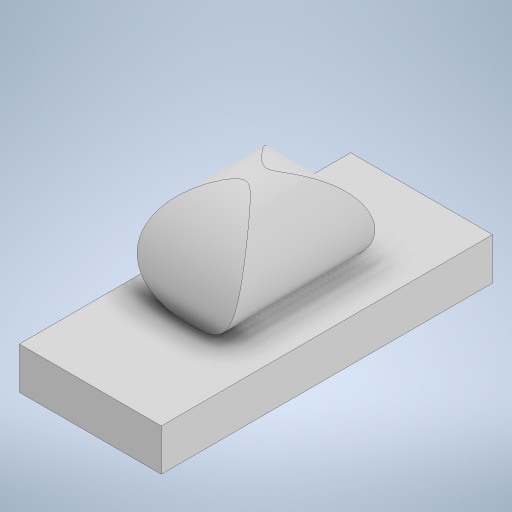
# Autodesk Inventor part: ball transfer unit
Saved by Autodesk Inventor 2023 (Build 270158000, 158)
## iProperties
Created: 2022-11-09
Part Number: ball transfer unit
Material: Generic
Document SubType Name: Modeling
Designer: cheng
Density: 1 g/cm^3
Appearance: Default
Author: cheng
Autodesk Inventor part; units mm, degrees
ref_plane "YZ Plane" through (0, 0, 0) normal (1, 0, 0) x (0, 1, 0)
ref_plane "XZ Plane" through (0, 0, 0) normal (0, 1, 0) x (-1, 0, 0)
ref_plane "XY Plane" through (0, 0, 0) normal (0, 0, 1) x (1, 0, 0)
sketch "Sketch1" plane through (0, 0, 0) normal (0, 1, 0) x (-1, 0, 0)
  line L0 (15, -35) -> (-15, -35)
  line L1 (-15, -35) -> (-15, 35)
  line L2 (-15, 35) -> (15, 35)
  line L3 (15, 35) -> (15, -35)
  line L4 (15, -35) -> (-15, 35) construction
  line L5 (-15, -35) -> (15, 35) construction
  point P0 (0, 0)
  dimension "d0" = 30
  dimension "d1" = 70
  constraints: 12 end point, 2 midpoint, 2 parallel, 1 horizontal, 1 perpendicular
  measures "d0" distance of L0.start L0.end
  measures "d1" distance of L2.end L0.start
extrude "Extrusion1" add sketch "Sketch1" along normal blind 30
sketch "Sketch2" plane through (15, 0, 35) normal (1, 0, 0) x (0, 0, -1)
  circle A0 centre (35, 15.1375) radius 14.909
  line L0 (0, 0) -> (0, 30) projected
  line L1 (0, 8.8455) -> (70, 8.8455)
  line L2 (0, 30) -> (70, 30) projected
  line L3 (0, 0) -> (70, 0) projected
  line L4 (70, 0) -> (70, 30) projected
  point P0 (35, 0)
  point P1 (36.1767, 30)
  point P2 (21.4837, 8.8455)
  point P3 (33.8233, 30)
  point P4 (48.5163, 8.8455)
  constraints: 2 end point, 2 point on line, 1 centre point, 1 horizontal, 1 perpendicular
extrude "Extrusion2" cut sketch "Sketch2" against normal blind 30 contours A0 L2 L4 L1 | A0 L1 L0 L2
sketch "Sketch3" plane through (-15, 0, 35) normal (0, 0, 1) x (1, 0, 0)
  circle A0 centre (15, 19.3194) radius 10.5597
  line L0 (0, 30) -> (0, 8.8455) projected
  line L1 (0, 30) -> (30, 30) projected
  line L2 (30, 8.8455) -> (30, 30) projected
  line L3 (30, 8.8455) -> (0, 8.8455) projected
  point P0 (15, 0)
  point P1 (13.6563, 8.8455)
  point P2 (16.3437, 8.8455)
  constraints: 1 centre point
extrude "Extrusion3" cut sketch "Sketch3" against normal blind 77 contours A0 L3 L0 L1 L2
body "Solid1"
